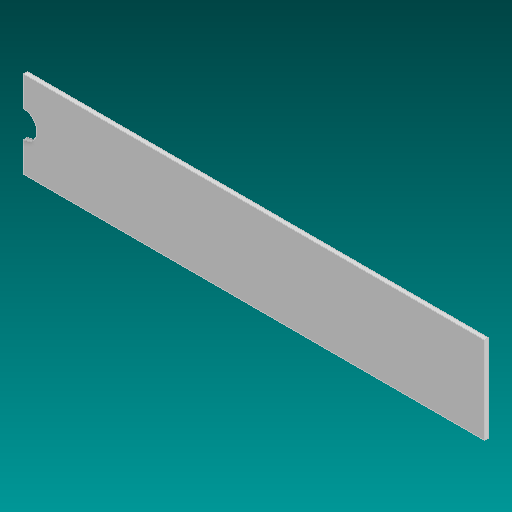
# Autodesk Inventor part: Part5
Saved by Autodesk Inventor 2020 (Build 240168000, 168)
## iProperties
Created: 2022-11-14
Part Number: Part5
Material: 一般
Document SubType Name: Modeling
Designer: Administrator
Density: 1 g/cm^3
Appearance: 既定
Author: Administrator
Autodesk Inventor part; units mm, degrees
ref_plane "YZ Plane" through (0, 0, 0) normal (1, 0, 0) x (0, 1, 0)
ref_plane "XZ Plane" through (0, 0, 0) normal (0, 1, 0) x (-1, 0, 0)
ref_plane "XY Plane" through (0, 0, 0) normal (0, 0, 1) x (1, 0, 0)
sketch "スケッチ1" plane through (0, 0, 0) normal (0, 0, 1) x (1, 0, 0)
  circle A0 centre (35.0095, -3.189) radius 22.5 projected
  circle A1 centre (35.0095, -3.189) radius 5 projected
  circle A2 centre (88.6134, 158.1387) radius 17.5
  line L0 (88.6134, 175.6387) -> (14.3927, 5.8219)
  line L1 (35.6723, -25.6792) -> (104.9163, 151.7773)
  line L2 (35.0095, -3.189) -> (35.0095, 12.811)
  line L3 (35.0095, 12.811) -> (205.0095, 12.811)
  line L4 (205.0095, 12.811) -> (205.0095, -19.189)
  line L5 (205.0095, -19.189) -> (35.0095, -19.189)
  line L6 (35.0095, -19.189) -> (35.0095, 12.811)
  circle A3 centre (88.6134, 158.1387) radius 5
  point P0 (0, 0)
  point P1 (35.0095, 1.811)
  point P2 (35.0095, -8.189)
  point P3 (205.0095, -8.189)
  point P4 (205.0095, 1.811)
  dimension "d0" = 35
  dimension "d1" = 170
  dimension "d4" = 16
  dimension "d5" = 170
  dimension "d6" = 32
  dimension "d7" = 10
  constraints: 14 end point, 4 point on circle, 2 centre point, 2 parallel, 2 tangent, 1 coincident, 1 horizontal, 1 perpendicular, 1 vertical
  measures "d0" diameter of A2
  measures "d1" distance of A2.centre A0.centre
  measures "d4" distance of L2.start L2.end
  measures "d5" distance of L4.end L5.end
  measures "d6" distance of L3.end L4.end
  measures "d7" diameter of A3
extrude "押し出し1" add sketch "スケッチ1" along normal blind 1.5 contours L5 L1 L3 A0 | A0 L3 L4 L5 | L5 L6 A1 L2 L3 L1
